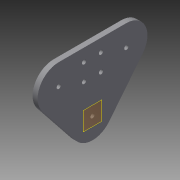
# Autodesk Inventor part: Arm_Base-SquareBar-Rev3
Saved by Autodesk Inventor 2015 (Build 190159000, 159)
## iProperties
Created: 2017-01-08
Part Number: Arm_Base-SquareBar-Rev3
Material: Generic
Document SubType Name: Modeling
Designer: Guy
Density: 1 g/cm^3
Appearance: Default
Author: Guy
Autodesk Inventor part; units mm, degrees
ref_plane "YZ Plane" through (0, 0, 0) normal (1, 0, 0) x (0, 1, 0)
ref_plane "XZ Plane" through (0, 0, 0) normal (0, 1, 0) x (-1, 0, 0)
ref_plane "XY Plane" through (0, 0, 0) normal (0, 0, 1) x (1, 0, 0)
sketch "Sketch1" plane through (0, 0, 0) normal (1, 0, 0) x (0, 1, 0)
  arc A0 (75.1, 40) -> (34.5017, 59.5369) centre (50.1, 40) ccw
  arc A1 (34.5017, -59.5369) -> (75.1, -40) centre (50.1, -40) ccw
  arc A2 (-15.5983, 19.5369) -> (-15.5983, -19.5369) centre (0, 0) ccw
  line L0 (34.5017, 59.5369) -> (-15.5983, 19.5369)
  line L1 (-15.5983, -19.5369) -> (34.5017, -59.5369)
  line L2 (75.1, -40) -> (75.1, 40)
  dimension "d0" = 80
  dimension "d1" = 50.1
  dimension "d2" = 50.1
  dimension "d3" = 40
  dimension "d4" = 50
  dimension "d5" = 50
  dimension "d6" = 50
  constraints: 6 end point, 6 point on circle, 6 tangent, 3 centre point, 1 coincident
  measures "d0" distance of A0.centre A1.centre
  measures "d1" horizontal distance of point (0, 0) A0.centre
  measures "d2" horizontal distance of point (0, 0) A1.centre
  measures "d3" vertical distance of point (0, 0) A1.centre
  measures "d4" diameter of A0
  measures "d5" diameter of A1
  measures "d6" diameter of A2
ref_plane "Work Plane1" through (6, 0, 0) normal (1, 0, 0) x (0, 0, -1)
sketch "Sketch2" plane through (6, 0, 0) normal (1, 0, 0) x (0, 0, -1)
  circle A0 centre (-40, 50.1) radius 2.5
  circle A1 centre (40, 50.1) radius 2.5
  circle A2 centre (0, 0) radius 2.5
  arc A3 (-19.5369, -15.5983) -> (19.5369, -15.5983) centre (0, 0) ccw projected
  line L0 (19.5369, -15.5983) -> (59.5369, 34.5017) projected
  arc A4 (59.5369, 34.5017) -> (40, 75.1) centre (40, 50.1) ccw projected
  line L1 (40, 75.1) -> (-40, 75.1) projected
  arc A5 (-40, 75.1) -> (-59.5369, 34.5017) centre (-40, 50.1) ccw projected
  line L2 (-59.5369, 34.5017) -> (-19.5369, -15.5983) projected
  dimension "d9" = 5
  dimension "d10" = 5
  dimension "d11" = 5
  constraints: 3 centre point, 3 coincident
  measures "d9" diameter of A0
  measures "d10" diameter of A1
  measures "d11" diameter of A2
ref_plane "Work Plane2" through (6, 0, 0) normal (1, 0, 0) x (0, 0, -1)
sketch "Sketch3" plane through (6, 0, 0) normal (1, 0, 0) x (0, 0, -1)
  circle A0 centre (40, 50.1) radius 2.5 projected
  circle A1 centre (-40, 50.1) radius 2.5 projected
  circle A2 centre (0, 0) radius 2.5 projected
  arc A3 (-19.5369, -15.5983) -> (19.5369, -15.5983) centre (0, 0) ccw projected
  line L0 (19.5369, -15.5983) -> (59.5369, 34.5017) projected
  arc A4 (59.5369, 34.5017) -> (40, 75.1) centre (40, 50.1) ccw projected
  line L1 (40, 75.1) -> (-40, 75.1) projected
  arc A5 (-40, 75.1) -> (-59.5369, 34.5017) centre (-40, 50.1) ccw projected
  line L2 (-59.5369, 34.5017) -> (-19.5369, -15.5983) projected
  circle A6 centre (-10, 40.1) radius 2.5
  circle A7 centre (10, 40.1) radius 2.5
  circle A8 centre (10, 60.1) radius 2.5
  circle A9 centre (-10, 60.1) radius 2.5
  dimension "d14" = 5
  dimension "d15" = 5
  dimension "d16" = 5
  dimension "d17" = 5
  dimension "d18" = 20
  dimension "d19" = 20
  dimension "d20" = 20
  dimension "d21" = 20
  dimension "d22" = 15
  dimension "d24" = 10
  dimension "d25" = 15
  dimension "d28" = 10
  constraints: 4 centre point
  measures "d14" diameter of A8
  measures "d15" diameter of A9
  measures "d16" diameter of A7
  measures "d17" diameter of A6
  measures "d18" distance of A8.centre A9.centre
  measures "d19" distance of A6.centre A7.centre
  measures "d20" distance of A7.centre A8.centre
  measures "d21" distance of A6.centre A9.centre
  measures "d22" distance from line of L1 A9.centre
  measures "d24" horizontal distance of A2.centre A8.centre
  measures "d25" distance from line of L1 A8.centre
  measures "d28" horizontal distance of A7.centre point (0, 0)
extrude "Extrusion4" add sketch "Sketch1" along normal blind 6
extrude "Extrusion5" cut sketch "Sketch3" against normal up to next contours A6 | A7 | A8 | A9
extrude "Extrusion6" cut sketch "Sketch2" against normal up to next contours A0 | A1 | A2
body "Solid1"
